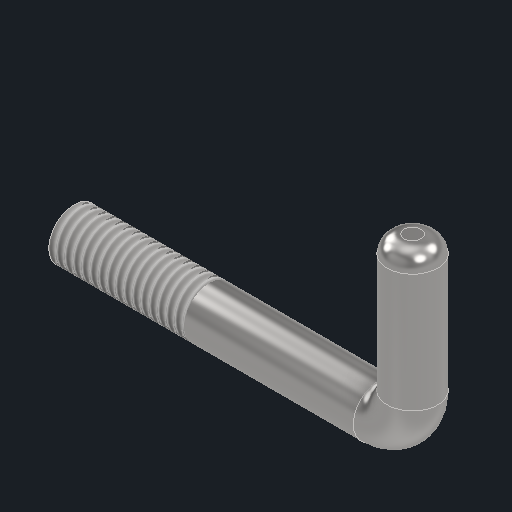
# Autodesk Inventor part: Lock Handel
Saved by Autodesk Inventor 2027.1 (Build 311270010, 270A)
## iProperties
Created: 2025-09-16
Part Number: Lock Handel
Material: Stainless Steel
Document SubType Name: Modeling
Designer: SD
Density: 8 g/cm^3
Appearance: Semi-Polished
Mass: 1.60351 g
Surface Area: 2.843 cm^2
Volume: 0.204268 cm^3
Project: Automatic Tea Steeping mechanism
BOM-Mass: 0.00160
BOM-Area: 0.000
Length: 35.000 mm
Diameter: 3.000 mm
Procurement: Fabricate - 1st round
Build Stage: 1
Preferred Material: 304 Stainless Steel
Author: SD
Title: Lock Handel
Autodesk Inventor part; units mm, degrees
ref_plane "YZ Plane" through (0, 0, 0) normal (1, 0, 0) x (0, 1, 0)
ref_plane "XZ Plane" through (0, 0, 0) normal (0, 1, 0) x (-1, 0, 0)
ref_plane "XY Plane" through (0, 0, 0) normal (0, 0, 1) x (1, 0, 0)
sketch "Sketch2" plane through (0, 0, 0) normal (0, 1, 0) x (-1, 0, 0)
  circle A0 centre (0, 0) radius 1.5
  dimension "Diameter" = 3
  constraints: 1 centre point, 1 coincident
  measures "Diameter" diameter of A0
sketch "Sketch1" plane through (0, 0, 0) normal (0, 0, 1) x (1, 0, 0)
  line L0 (0, 0) -> (0, -8)
  line L1 (-2, -10) -> (-20, -10)
  arc A0 (-2, -10) -> (0, -8) centre (-2, -8) ccw
  point P0 (0, -10)
  dimension "d0" = 10
  dimension "d1" = 20
  dimension "d2" = 2
  constraints: 4 end point, 2 point on circle, 2 point on line, 2 tangent, 1 centre point, 1 perpendicular, 1 vertical
  measures "d0" distance of L0.start point (0, -10)
  measures "d1" distance of point (0, -10) L1.end
  measures "d2" radius of A0
sweep "Sweep1" add profiles "Sketch2" path "Sketch1" path curves L0 A0 L1
thread "Thread1"
fillet "Fillet1" radius 1 1 edges at (1.5, 0, 0)
equation "\"Length\" = 35"
body "Solid1"
